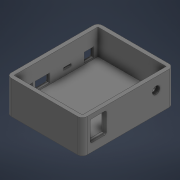
# Autodesk Inventor part: Case Proyecto IOT
Saved by Autodesk Inventor 2021 (Build 250183000, 183)
## iProperties
Created: 2021-03-29
Part Number: Case Proyecto IOT
Material: Genérico
Document SubType Name: Modeling
Designer: grego
Density: 1 g/cm^3
Appearance: Valor por defecto
Author: grego
Autodesk Inventor part; units mm, degrees
ref_plane "YZ Plane" through (0, 0, 0) normal (1, 0, 0) x (0, 1, 0)
ref_plane "XZ Plane" through (0, 0, 0) normal (0, 1, 0) x (-1, 0, 0)
ref_plane "XY Plane" through (0, 0, 0) normal (0, 0, 1) x (1, 0, 0)
sketch "Boceto1" plane through (0, 0, 0) normal (0, 1, 0) x (-1, 0, 0)
  line L0 (0, 0) -> (80.1, 0)
  line L1 (80.1, 0) -> (80.1, -96.5)
  line L2 (80.1, -96.5) -> (0, -96.5)
  line L3 (0, -96.5) -> (0, 0)
  dimension "d0" = 80.1
  dimension "d1" = 96.5
  constraints: 8 end point, 2 parallel, 1 horizontal, 1 perpendicular
  measures "d0" distance of L1.end L2.end
  measures "d1" distance of L0.end L1.end
extrude "Extrusión1" add sketch "Boceto1" along normal blind 8
sketch "Boceto2" plane through (0, 8, 0) normal (0, 1, 0) x (1, 0, 0)
  line L0 (-80.1, 96.5) -> (-80.1, 0) projected
  line L1 (-80.1, 0) -> (0, 0) projected
  line L2 (-80.1, 96.5) -> (0, 96.5)
  line L3 (0, 96.5) -> (0, 0)
  line L4 (0, 0) -> (-80.1, 0)
  line L5 (-80.1, 0) -> (-80.1, 96.5)
  line L6 (-76.1, 92.5) -> (-4, 92.5)
  line L7 (-4, 92.5) -> (-4, 4)
  line L8 (-4, 4) -> (-76.1, 4)
  line L9 (-76.1, 4) -> (-76.1, 92.5)
  dimension "d4" = 4
  dimension "d5" = 4
  dimension "d6" = 4
  dimension "d7" = 4
  constraints: 16 end point, 4 parallel, 2 horizontal, 2 perpendicular
  measures "d4" distance between parallel lines of L6 L2
  measures "d5" distance between parallel lines of L9 L0
  measures "d6" distance between parallel lines of L3 L7
  measures "d7" distance between parallel lines of L1 L8
extrude "Extrusión2" add sketch "Boceto2" along normal blind 27.02
fillet "Empalme1" radius 5 4 edges at (-80.1, 17.51, -96.5) (-80.1, 17.51, 0) (0, 17.51, 0) (0, 17.51, -96.5)
sketch "Boceto16" plane through (0, 0, -5) normal (1, 0, 0) x (0, 0, -1)
  circle A0 centre (72.76, 22.606) radius 4
  line L0 (14.98, 29.606) -> (19.28, 29.606) projected
  line L1 (4.38, 29.606) -> (8.68, 29.606) projected
  line L2 (4.18, 29.806) -> (4.18, 9.606) projected
  line L3 (19.48, 9.606) -> (19.48, 29.806) projected
  line L4 (4.38, 9.606) -> (19.28, 9.606) projected
  line L5 (4.18, 29.606) -> (19.48, 29.606)
  line L6 (19.48, 29.606) -> (19.48, 9.606)
  line L7 (19.48, 9.606) -> (4.18, 9.606)
  line L8 (4.18, 9.606) -> (4.18, 29.606)
  point P0 (-5, 0)
  point P1 (4.18, 9.606)
  point P2 (8.68, 29.606)
  dimension "d50" = 8
  constraints: 8 end point, 2 parallel, 1 centre point, 1 horizontal, 1 perpendicular, 1 point on line
  measures "d50" diameter of A0
extrude "Extrusión11" cut sketch "Boceto16" against normal blind 10
sketch "Boceto17" plane through (-80.1, 0, -91.5) normal (-1, 0, 0) x (0, 0, 1)
  line L0 (67.71, 18.606) -> (67.71, 9.606) projected
  line L1 (82.71, 18.606) -> (67.71, 18.606) projected
  line L2 (82.71, 18.606) -> (82.71, 9.606) projected
  line L3 (82.71, 9.606) -> (67.71, 9.606) projected
  line L4 (65.14, 18.606) -> (65.14, 9.606) projected
  line L5 (65.14, 18.606) -> (50.14, 18.606) projected
  line L6 (50.14, 18.606) -> (50.14, 9.606) projected
  line L7 (65.14, 9.606) -> (50.14, 9.606) projected
  line L8 (13.54, 9.606) -> (13.54, 17.606) projected
  line L9 (13.54, 17.606) -> (13.54, 19.273) projected
  line L10 (3.54, 19.273) -> (13.54, 19.273) projected
  line L11 (3.54, 9.606) -> (3.54, 17.606) projected
  line L12 (-1, 9.606) -> (87.5, 9.606) projected
  line L13 (50.14, 18.606) -> (65.14, 18.606)
  line L14 (65.14, 18.606) -> (65.14, 9.606)
  line L15 (65.14, 9.606) -> (50.14, 9.606)
  line L16 (50.14, 9.606) -> (50.14, 18.606)
  line L17 (67.71, 18.606) -> (82.71, 18.606)
  line L18 (82.71, 18.606) -> (82.71, 9.606)
  line L19 (82.71, 9.606) -> (67.71, 9.606)
  line L20 (67.71, 9.606) -> (67.71, 18.606)
  line L21 (13.54, 19.273) -> (3.54, 19.273)
  line L22 (3.54, 19.273) -> (3.54, 9.606)
  line L23 (3.54, 9.606) -> (13.54, 9.606)
  line L24 (13.54, 9.606) -> (13.54, 19.273)
  line L25 (27.7762, 13.6111) -> (34.9176, 13.6111)
  line L26 (35.4176, 14.1111) -> (35.4176, 15.456)
  line L27 (34.9176, 15.956) -> (27.7762, 15.956)
  line L28 (27.2762, 15.456) -> (27.2762, 14.1111)
  arc A0 (27.7762, 15.956) -> (27.2762, 15.456) centre (27.7762, 15.456) ccw
  arc A1 (27.2762, 14.1111) -> (27.7762, 13.6111) centre (27.7762, 14.1111) ccw
  arc A2 (34.9176, 13.6111) -> (35.4176, 14.1111) centre (34.9176, 14.1111) ccw
  arc A3 (35.4176, 15.456) -> (34.9176, 15.956) centre (34.9176, 15.456) ccw
  point P0 (91.5, 0)
  point P1 (3.54, 17.606)
  dimension "d56" = 0.5
  constraints: 32 end point, 8 parallel, 8 point on circle, 8 tangent, 4 centre point, 4 perpendicular, 3 equal radius, 3 horizontal
  measures "d56" radius of A0
extrude "Extrusión12" cut sketch "Boceto17" against normal blind 10
sketch "Boceto18" plane through (-80.1, 0, -91.5) normal (-1, 0, 0) x (0, 0, 1)
  line L0 (27.7762, 15.956) -> (34.9176, 15.956) projected
  arc A0 (27.7762, 15.956) -> (27.2762, 15.456) centre (27.7762, 15.456) ccw projected
  line L1 (27.2762, 14.1111) -> (27.2762, 15.456) projected
  arc A1 (27.2762, 14.1111) -> (27.7762, 13.6111) centre (27.7762, 14.1111) ccw projected
  line L2 (34.9176, 13.6111) -> (27.7762, 13.6111) projected
  arc A2 (34.9176, 13.6111) -> (35.4176, 14.1111) centre (34.9176, 14.1111) ccw projected
  line L3 (35.4176, 15.456) -> (35.4176, 14.1111) projected
  arc A3 (35.4176, 15.456) -> (34.9176, 15.956) centre (34.9176, 15.456) ccw projected
  line L4 (34.9176, 16.956) -> (27.7762, 16.956)
  arc A4 (27.7762, 16.956) -> (26.2762, 15.456) centre (27.7762, 15.456) ccw
  line L5 (26.2762, 15.456) -> (26.2762, 14.1111)
  arc A5 (26.2762, 14.1111) -> (27.7762, 12.6111) centre (27.7762, 14.1111) ccw
  line L6 (27.7762, 12.6111) -> (34.9176, 12.6111)
  arc A6 (34.9176, 12.6111) -> (36.4176, 14.1111) centre (34.9176, 14.1111) ccw
  line L7 (36.4176, 14.1111) -> (36.4176, 15.456)
  arc A7 (36.4176, 15.456) -> (34.9176, 16.956) centre (34.9176, 15.456) ccw
  line L8 (13.54, 19.273) -> (13.54, 9.606) projected
  line L9 (3.54, 19.273) -> (13.54, 19.273) projected
  line L10 (3.54, 9.606) -> (3.54, 19.273) projected
  line L11 (13.54, 9.606) -> (3.54, 9.606) projected
  line L12 (65.14, 9.606) -> (50.14, 9.606) projected
  line L13 (50.14, 9.606) -> (50.14, 18.606) projected
  line L14 (50.14, 18.606) -> (65.14, 18.606) projected
  line L15 (65.14, 18.606) -> (65.14, 9.606) projected
  line L16 (67.71, 18.606) -> (82.71, 18.606) projected
  line L17 (67.71, 9.606) -> (67.71, 18.606) projected
  line L18 (82.71, 18.606) -> (82.71, 9.606) projected
  line L19 (82.71, 9.606) -> (67.71, 9.606) projected
  line L20 (14.54, 18.273) -> (14.54, 10.606)
  line L21 (12.54, 8.606) -> (4.54, 8.606)
  line L22 (2.54, 10.606) -> (2.54, 18.273)
  line L23 (4.54, 20.273) -> (12.54, 20.273)
  line L24 (64.14, 19.606) -> (51.14, 19.606)
  line L25 (49.14, 17.606) -> (49.14, 10.606)
  line L26 (51.14, 8.606) -> (64.14, 8.606)
  line L27 (66.14, 10.606) -> (66.14, 17.606)
  line L28 (81.71, 19.606) -> (68.71, 19.606)
  line L29 (66.71, 17.606) -> (66.71, 10.606)
  line L30 (68.71, 8.606) -> (81.71, 8.606)
  line L31 (83.71, 10.606) -> (83.71, 17.606)
  arc A8 (4.54, 20.273) -> (2.54, 18.273) centre (4.54, 18.273) ccw
  arc A9 (14.54, 18.273) -> (12.54, 20.273) centre (12.54, 18.273) ccw
  arc A10 (2.54, 10.606) -> (4.54, 8.606) centre (4.54, 10.606) ccw
  arc A11 (12.54, 8.606) -> (14.54, 10.606) centre (12.54, 10.606) ccw
  arc A12 (49.14, 10.606) -> (51.14, 8.606) centre (51.14, 10.606) ccw
  arc A13 (51.14, 19.606) -> (49.14, 17.606) centre (51.14, 17.606) ccw
  arc A14 (66.14, 17.606) -> (64.14, 19.606) centre (64.14, 17.606) ccw
  arc A15 (64.14, 8.606) -> (66.14, 10.606) centre (64.14, 10.606) ccw
  arc A16 (68.71, 19.606) -> (66.71, 17.606) centre (68.71, 17.606) ccw
  arc A17 (66.71, 10.606) -> (68.71, 8.606) centre (68.71, 10.606) ccw
  arc A18 (83.71, 17.606) -> (81.71, 19.606) centre (81.71, 17.606) ccw
  arc A19 (81.71, 8.606) -> (83.71, 10.606) centre (81.71, 10.606) ccw
  point P0 (91.5, 0)
  dimension "d62" = 1
  dimension "d65" = 1
  dimension "d66" = 1
  dimension "d67" = 1
  dimension "d68" = 2
  constraints: 32 end point, 32 point on circle, 24 tangent, 16 centre point, 11 equal radius, 16 other
  measures "d62" distance between parallel lines of L0 L4
  measures "d65" distance between parallel lines of L9 L23
  measures "d66" distance between parallel lines of L14 L24
  measures "d67" distance between parallel lines of L16 L28
  measures "d68" radius of A8
extrude "Extrusión13" cut sketch "Boceto18" against normal blind 2 contours A7 L7 A6 L6 A5 L5 A4 L4 | L8 L11 L10 L9 | L20 A11 L21 A10 L22 A8 L23 A9 | A14 L27 A15 L26 A12 L25 A13 L24 | A18 L31 A19 L30 A17 L29 A16 L28
sketch "Boceto19" plane through (-80.1, 0, -91.5) normal (-1, 0, 0) x (0, 0, 1)
  line L0 (5.1093, 25.2349) -> (7.6216, 25.2349)
  line L1 (7.6216, 25.2349) -> (7.6216, 24.5349)
  line L2 (7.6216, 24.5349) -> (5.3547, 24.5349)
  line L3 (5.1093, 25.2349) -> (4.6547, 25.2349)
  line L4 (5.175, 24.5349) -> (5.1093, 24.5349)
  line L5 (5.1093, 24.5349) -> (4.6547, 24.5349)
  line L6 (4.6547, 25.2349) -> (4.6547, 23.8349)
  arc A0 (4.6547, 21.2123) -> (5.3547, 23.8349) centre (5.9736, 22.265) ccw
  arc A1 (5.2018, 21.649) -> (5.6114, 23.1837) centre (5.9736, 22.265) ccw
  line L7 (5.3547, 24.5349) -> (5.3547, 23.8349)
  line L8 (5.2018, 21.649) -> (4.6547, 21.2123)
  line L9 (5.6114, 23.1837) -> (4.6547, 23.1837)
  line L10 (4.6547, 23.1837) -> (4.6547, 23.8349)
  line L11 (8.54, 23.5093) -> (9.5953, 20.5268)
  line L12 (9.5953, 20.5268) -> (10.8465, 20.5268)
  line L13 (4.54, 20.273) -> (12.54, 20.273) projected
  line L14 (10.8465, 20.5268) -> (11.9556, 23.5093)
  line L15 (11.9556, 23.5093) -> (11.2556, 23.5093)
  line L16 (11.2556, 23.5093) -> (10.2993, 20.9376)
  line L17 (10.2993, 20.9376) -> (9.9991, 20.9376)
  line L18 (9.9991, 20.9376) -> (9.0891, 23.5093)
  line L19 (9.0891, 23.5093) -> (8.54, 23.5093)
  point P0 (91.5, 0)
  dimension "d69" = 0.7
  dimension "d70" = 0.7
  dimension "d73" = 0.7
  dimension "d76" = 0.7
  constraints: 38 end point, 6 parallel, 4 point on circle, 3 horizontal, 3 perpendicular, 2 centre point, 2 vertical, 1 point on line, 1 other
  measures "d69" distance of L0.end L1.end
  measures "d70" distance of L2.end L7.end
  measures "d73" radial gap between concentric circles of A0 A1
  measures "d76" distance of L14.end L15.end
emboss "Repujado1" sketch "Boceto19" operation add depth 0.3 direction (1, 0, 0)
sketch "Boceto20" plane through (0, 0, -5) normal (1, 0, 0) x (0, 0, -1)
  line L0 (19.48, 29.606) -> (19.48, 9.606) projected
  line L1 (4.18, 29.606) -> (19.48, 29.606) projected
  line L2 (4.18, 9.606) -> (4.18, 29.606) projected
  line L3 (19.48, 9.606) -> (4.18, 9.606) projected
  line L4 (20.48, 10.606) -> (20.48, 28.606)
  line L5 (18.48, 30.606) -> (5.18, 30.606)
  line L6 (3.18, 28.606) -> (3.18, 10.606)
  line L7 (5.18, 8.606) -> (18.48, 8.606)
  arc A0 (5.18, 30.606) -> (3.18, 28.606) centre (5.18, 28.606) ccw
  arc A1 (20.48, 28.606) -> (18.48, 30.606) centre (18.48, 28.606) ccw
  arc A2 (18.48, 8.606) -> (20.48, 10.606) centre (18.48, 10.606) ccw
  arc A3 (3.18, 10.606) -> (5.18, 8.606) centre (5.18, 10.606) ccw
  point P0 (-5, 0)
  point P1 (20.48, 8.606)
  point P2 (20.48, 30.606)
  point P3 (3.18, 30.606)
  point P4 (3.18, 8.606)
  dimension "d77" = 1
  dimension "d80" = 2
  constraints: 8 end point, 8 point on circle, 8 point on line, 8 tangent, 4 centre point, 3 equal radius, 3 other
  measures "d77" distance between parallel lines of L0 L4
  measures "d80" radius of A0
extrude "Extrusión14" cut sketch "Boceto20" against normal blind 2
